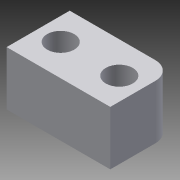
# Autodesk Inventor part: yCarMid_c
Saved by Autodesk Inventor 2013 (Build 170138000, 138)
## iProperties
Created: 2015-01-14
Part Number: yCarMid_c
Material: Generic
Document SubType Name: Modeling
Designer: dzban
Density: 1 g/cm^3
Author: dzban
Autodesk Inventor part; units mm, degrees
ref_plane "YZ Plane" through (0, 0, 0) normal (1, 0, 0) x (0, 1, 0)
ref_plane "XZ Plane" through (0, 0, 0) normal (0, 1, 0) x (-1, 0, 0)
ref_plane "XY Plane" through (0, 0, 0) normal (0, 0, 1) x (1, 0, 0)
sketch "Sketch1" plane through (0, 0, 0) normal (0, 0, 1) x (1, 0, 0)
  circle A0 centre (-9, 3.5) radius 1.5
  circle A1 centre (-2.5, 3.5) radius 1.5
  line L0 (0, 0) -> (-11.5, 0)
  line L1 (0, 5) -> (0, 0)
  arc A2 (0, 5) -> (-2, 7) centre (-2, 5) ccw
  line L2 (-11.5, 7) -> (-2, 7)
  line L3 (-11.5, 0) -> (-11.5, 7)
  constraints: 8 end point, 3 centre point, 2 point on circle
extrude "Extrusion1" add sketch "Sketch1" along normal blind 6
body "Solid1"
